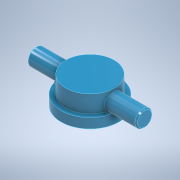
# Autodesk Inventor part: EChem _S200 Cap Top
Saved by Autodesk Inventor 2021 (Build 250183000, 183)
## iProperties
Created: 2020-07-06
Part Number: EChem _S200 Cap Top
Material: Generic
Document SubType Name: Modeling
Designer: jgray
Density: 1 g/cm^3
Appearance: Default
Author: jgray
Autodesk Inventor part; units mm, degrees
ref_plane "YZ Plane" through (0, 0, 0) normal (1, 0, 0) x (0, 1, 0)
ref_plane "XZ Plane" through (0, 0, 0) normal (0, 1, 0) x (-1, 0, 0)
ref_plane "XY Plane" through (0, 0, 0) normal (0, 0, 1) x (1, 0, 0)
sketch "Sketch1" plane through (0, 0, 0) normal (0, 1, 0) x (-1, 0, 0)
  circle A0 centre (0, 0) radius 11
  dimension "d0" = 22
  constraints: 1 centre point, 1 coincident
  measures "d0" diameter of A0
extrude "Extrusion1" add sketch "Sketch1" along normal blind 3.9
sketch "Sketch2" plane through (0, 3.9, 0) normal (0, 1, 0) x (1, 0, 0)
  circle A0 centre (0, 0) radius 9.2
  dimension "d3" = 18.4
  constraints: 1 centre point, 1 coincident
  measures "d3" diameter of A0
extrude "Extrusion2" add sketch "Sketch2" along normal blind 6.55
sketch "Sketch3" plane through (0, 0, 0) normal (0, 0, 1) x (1, 0, 0)
  line L0 (18.8479, 6.1) -> (-23.7231, 6.1)
  line L1 (11, 0) -> (-11, 0) projected
  line L2 (20.75, 6.1) -> (-20.75, 6.1)
  line L3 (-20.75, 6.1) -> (-20.75, 9.3)
  line L4 (-20.75, 9.3) -> (20.75, 9.3)
  line L5 (20.75, 9.3) -> (20.75, 6.1)
  line L6 (9.2, 10.45) -> (-9.2, 10.45) construction
  line L7 (0, 10.45) -> (0, -1.5119) construction
  point P0 (0, 0)
  point P1 (0, 9.3)
  dimension "d6" = 6.1
  dimension "d7" = 41.5
  dimension "d8" = 3.2
  constraints: 12 end point, 2 horizontal, 2 midpoint, 2 parallel, 2 point on line, 1 perpendicular, 1 vertical
  measures "d6" distance between parallel lines of L0 L1
  measures "d7" distance of L3.end L4.end
  measures "d8" distance of L2.end L3.end
revolve "Revolution1" add sketch "Sketch3" angle 360 about axis through (18.8479, 6.1, 0) along (1, 0, 0)
chamfer "Chamfer1" distance 0.5 angle 45 2 edges at (-20.75, 2.9, 0) (20.75, 2.9, 0)
fillet "Fillet1" radius 0.5 4 edges at (9.8267, 3.9, 2.3238) (9.8267, 3.9, -2.3238) (-9.8267, 3.9, 2.3238) (-9.8267, 3.9, -2.3238)
chamfer "Chamfer2" distance 0.2 angle 45 1 edges at (11, 0, 0)
body "Solid1"
